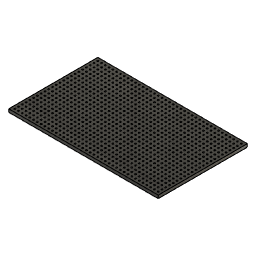
protoboard (Autodesk Fusion 360 design; units mm, degrees)
Autodesk Fusion 360 part; units mm, degrees
sketch "Esquisse1" plane through (0, 0, 0) normal (0, 0, 1) x (1, 0, 0)
  line L0 (49.5, 29.5) -> (-49.5, 29.5)
  line L1 (-49.5, 29.5) -> (-49.5, -29.5)
  line L2 (-49.5, -29.5) -> (49.5, -29.5)
  line L3 (49.5, -29.5) -> (49.5, 29.5)
  line L4 (0, 29.5) -> (0, -29.5) construction
  dimension "d1" = 59
  dimension "d2" = 99
  constraint horizontal L0
  constraint perpendicular L0 L1
  constraint parallel L0 L2
  constraint parallel L1 L3
  constraint midpoint L0 L4.start
  constraint midpoint L2 L4.end
  constraint midpoint origin L4
  measures "d1" distance of L0 L2
  measures "d2" distance of L1 L3
extrude "Extrusion1" add sketch "Esquisse1" along normal mid plane 2
sketch "Esquisse2" plane through (0, 0, 1) normal (0, 0, 1) x (-1, 0, 0)
  line L0 (-49.5, 29.5) -> (-49.5, -29.5)
  line L1 (-49.5, -29.5) -> (49.5, -29.5)
  line L2 (49.5, -29.5) -> (49.5, 29.5)
  line L3 (49.5, 29.5) -> (-49.5, 29.5)
  line L4 (49.5, -27.5) -> (47.5, -27.5) construction
  line L5 (47.5, -27.5) -> (47.5, -29.5) construction
  circle A0 centre (47.5, -27.5) radius 0.5
  point P0 (48, -27.5)
  point P1 (47.5, -28)
  dimension "d5" = 1
  dimension "d15" = 1.5
  dimension "d16" = 1.5
  constraint coincident L2 L4.start
  constraint perpendicular L2 L4
  constraint coincident L1 L5.end
  constraint perpendicular L1 L5
  constraint coincident L4.end L5.start
  constraint coincident A0 P0
  constraint coincident L4 P0
  constraint coincident L5 P1
  constraint coincident A0 P1
  measures "d5" diameter of A0
  measures "d15" distance of L4.start P0
  measures "d16" distance of L5.end P1
extrude "Extrusion2" cut sketch "Esquisse2" against normal up to surface (2 mm away) contours A0
pattern_linear "hole_grid" count 39 spacing 2.5 along (1, 0, 0) count 23 spacing 2.5 along (0, -1, 0) of "Extrusion2"
equation "d1 = plate_width"
equation "d2 = plate_length"
equation "d3 = plate_thickness"
equation "d5 = hole_size"
equation "plate_width = 59 mm"
equation "plate_length = 99 mm"
equation "min_hole_h_offset = 1.5 mm" comment "Minimum horizontal distance of the hole grid and the sides"
equation "min_hole_v_offset = 1.5 mm" comment "Minimum vertical distance of the hole grid and the sides"
equation "hole_size = 1 mm"
equation "d15 = min_hole_h_offset + _hole_h_offset_surplus / 2"
equation "d16 = min_hole_v_offset + _hole_v_offset_surplus / 2"
equation "hole_h_spacing = min_hole_h_offset" comment "Horizontal distance between holes"
equation "hole_v_spacing = min_hole_v_offset" comment "Vertical distance between holes"
equation "_nb_h_holes = floor(( plate_length - 2 * min_hole_h_offset + hole_h_spacing ) / ( hole_size + hole_h_spacing ))" comment "Not intended to be changed"
equation "_nb_v_holes = floor(( plate_width - 2 * min_hole_v_offset + hole_v_spacing ) / ( hole_size + hole_v_spacing ))" comment "Not intended to be changed"
equation "d23 = _nb_h_holes"
equation "d24 = _nb_v_holes"
equation "d25 = hole_h_spacing + hole_size"
equation "d26 = hole_v_spacing + hole_size"
equation "_hole_h_offset_surplus = ( plate_length - 2 * min_hole_h_offset ) - ( _nb_h_holes * hole_size + ( _nb_h_holes - 1 ) * hole_h_spacing )" comment "Do not change! Used only for calculations (for centering of holes)"
equation "_hole_v_offset_surplus = ( plate_width - 2 * min_hole_v_offset ) - ( _nb_v_holes * hole_size + ( _nb_v_holes - 1 ) * hole_v_spacing )" comment "Do not change! Used only for calculations (for centering of holes)"
equation "plate_thickness = 2 mm"
named bodies: "protoboard"
